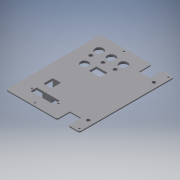
# Autodesk Inventor part: vrch2
Saved by Autodesk Inventor 2016 (Build 200138000, 138)
## iProperties
Created: 2015-11-06
Part Number: vrch2
Material: Generic
Document SubType Name: Modeling
Designer: Jufo
Density: 1 g/cm^3
Appearance: Default
Author: Jufo
Autodesk Inventor part; units mm, degrees
ref_plane "YZ Plane" through (0, 0, 0) normal (1, 0, 0) x (0, 1, 0)
ref_plane "XZ Plane" through (0, 0, 0) normal (0, 1, 0) x (-1, 0, 0)
ref_plane "XY Plane" through (0, 0, 0) normal (0, 0, 1) x (1, 0, 0)
sketch "Sketch1" plane through (0, 0, 0) normal (0, 1, 0) x (-1, 0, 0)
  line L0 (8.278, -23.2242) -> (24.278, -23.2242)
  line L1 (24.278, -23.2242) -> (24.278, 3.7758)
  line L2 (24.278, 3.7758) -> (48.278, 3.7758)
  line L3 (48.278, 3.7758) -> (48.278, -23.2242)
  line L4 (48.278, -23.2242) -> (88.278, -23.2242)
  line L5 (48.278, -23.2242) -> (136.1936, -23.2242)
  line L6 (136.1936, -23.2242) -> (136.1936, 142.7758)
  line L7 (136.1936, 142.7758) -> (48.278, 142.7758)
  line L8 (48.278, 142.7758) -> (48.278, 115.7758)
  line L9 (48.278, 115.7758) -> (24.278, 115.7758)
  line L10 (24.278, 115.7758) -> (24.278, 142.7758)
  line L11 (24.278, 142.7758) -> (24.278, 115.7758)
  line L12 (8.278, 142.7758) -> (24.278, 142.7758)
  line L13 (24.278, 142.7758) -> (8.278, 142.7758)
  line L14 (8.278, 142.7758) -> (8.278, -23.2242)
  line L15 (24.278, 3.7758) -> (24.278, -23.2242)
  circle A0 centre (11.278, -20.2242) radius 1.5
  circle A1 centre (11.278, -20.2242) radius 1.5
  circle A2 centre (11.278, 139.7758) radius 1.5
  circle A3 centre (11.278, 139.7758) radius 1.5
  circle A4 centre (91.278, -20.2242) radius 1.5
  circle A5 centre (91.278, -20.2242) radius 1.5
  circle A6 centre (91.278, 139.7758) radius 1.5
  circle A7 centre (91.278, 139.7758) radius 1.5
  line L16 (133.1936, 141.7758) -> (49.278, 141.7758)
  line L17 (49.278, 141.7758) -> (49.278, 114.7758)
  line L18 (49.278, 114.7758) -> (23.278, 114.7758)
  line L19 (23.278, 114.7758) -> (23.278, 141.7758)
  line L20 (8.278, 59.7758) -> (68.278, 59.7758)
  line L21 (133.1936, 141.7758) -> (133.1936, 59.7758)
  line L22 (23.278, 141.7758) -> (9.278, 141.7758)
  line L23 (9.278, 141.7758) -> (9.278, 59.7758)
  line L24 (133.1936, -22.2242) -> (49.278, -22.2242)
  line L25 (49.278, -22.2242) -> (49.278, 4.7758)
  line L26 (49.278, 4.7758) -> (23.278, 4.7758)
  line L27 (23.278, 4.7758) -> (23.278, -22.2242)
  line L28 (133.1936, -22.2242) -> (133.1936, 59.7758)
  line L29 (23.278, -22.2242) -> (9.278, -22.2242)
  line L30 (9.278, -22.2242) -> (9.278, 59.7758)
  point P0 (0, 0)
  point P1 (0, 0)
  dimension "d0" = 24
  dimension "d1" = 16
  dimension "d2" = 87.9156
  dimension "d3" = 166
  dimension "d4" = 3
  dimension "d5" = 27
  dimension "d6" = 1
  dimension "d8" = 1
  dimension "d9" = 1
  dimension "d10" = 1
  dimension "d11" = 1
  constraints: 62 end point, 13 perpendicular, 8 centre point, 6 symmetric about line, 5 point on line, 4 coincident, 3 horizontal, 2 parallel, 1 midpoint, 1 vertical
  measures "d0" distance of L8.end L9.end
  measures "d1" distance of L10.end L12.start
  measures "d2" distance of L6.end L7.end
  measures "d3" distance of L5.end L6.end
  measures "d4" distance between parallel lines of L6 L21
  measures "d5" distance of L7.end L8.end
  measures "d6" distance between parallel lines of L8 L17
  measures "d8" distance between parallel lines of L18 L9
  measures "d9" distance between parallel lines of L19 L10
  measures "d10" distance between parallel lines of L12 L22
  measures "d11" distance between parallel lines of L14 L23
extrude "Extrusion1" add sketch "Sketch1" along normal blind 2 contours L21 L28 L24 L25 L26 L27 L29 L30 L23 L22 L19 L18 L17 L16
sketch "Sketch2" plane through (0, 2, 0) normal (0, 1, 0) x (1, 0, 0)
  line L0 (-6.278, 25.2242) -> (-26.278, 25.2242)
  line L1 (-26.278, 25.2242) -> (-26.278, 2.2242)
  line L2 (-26.278, 2.2242) -> (-46.278, 2.2242)
  line L3 (-46.278, 2.2242) -> (-46.278, 25.2242)
  line L4 (-46.278, 25.2242) -> (-138.2936, 25.2242)
  line L5 (-133.1936, 22.2242) -> (-133.1936, -141.7758) projected
  line L6 (-133.1936, -59.7758) -> (-63.3349, -59.7758)
  line L7 (-138.2936, 25.2242) -> (-138.2936, -59.7758)
  line L8 (-6.278, 25.2242) -> (-6.278, -59.7758)
  line L9 (-9.278, -141.7758) -> (-9.278, 22.2242) projected
  line L10 (-9.278, 22.2242) -> (-23.278, 22.2242) projected
  line L11 (-23.278, 22.2242) -> (-23.278, -4.7758) projected
  line L12 (-23.278, -4.7758) -> (-49.278, -4.7758) projected
  line L13 (-49.278, -4.7758) -> (-49.278, 22.2242) projected
  line L14 (-49.278, 22.2242) -> (-133.1936, 22.2242) projected
  line L15 (-6.278, -144.7758) -> (-26.278, -144.7758)
  line L16 (-26.278, -144.7758) -> (-26.278, -121.7758)
  line L17 (-26.278, -121.7758) -> (-46.278, -121.7758)
  line L18 (-46.278, -121.7758) -> (-46.278, -144.7758)
  line L19 (-46.278, -144.7758) -> (-138.2936, -144.7758)
  line L20 (-6.278, -144.7758) -> (-6.278, -59.7758)
  line L21 (-138.2936, 25.2242) -> (-138.2936, -144.7758)
  circle A0 centre (-91.278, 20.2242) radius 1.5 projected
  circle A1 centre (-91.278, 20.2242) radius 1.5
  circle A2 centre (-91.278, -139.7758) radius 1.5 projected
  circle A3 centre (-91.278, -139.7758) radius 1.5
  circle A4 centre (-11.278, -139.7758) radius 1.5 projected
  circle A5 centre (-11.278, -139.7758) radius 1.5
  circle A6 centre (-11.278, 20.2242) radius 1.5
  point P0 (0, 0)
  dimension "d14" = 3
  dimension "d15" = 3
  dimension "d16" = 3
  dimension "d17" = 7
  dimension "d18" = 3
  dimension "d19" = 3
  dimension "d130" = 5.1
  constraints: 30 end point, 6 symmetric about line, 5 point on line, 4 centre point, 4 perpendicular, 3 coincident, 2 horizontal, 1 concentric, 1 midpoint, 1 parallel, 1 vertical
  measures "d14" distance between parallel lines of L8 L9
  measures "d15" distance between parallel lines of L0 L10
  measures "d16" distance between parallel lines of L1 L11
  measures "d17" distance between parallel lines of L12 L2
  measures "d18" distance between parallel lines of L13 L3
  measures "d19" distance between parallel lines of L4 L14
  measures "d130" distance between parallel lines of L5 L21
extrude "Extrusion2" add sketch "Sketch2" along normal blind 2
sketch "Sketch9" plane through (0, 4, 0) normal (0, 1, 0) x (1, 0, 0)
  line L0 (-26.278, -121.7758) -> (-6.278, -121.7758)
  line L1 (-6.278, -144.7758) -> (-6.278, 25.2242) projected
  line L2 (-26.278, 2.2242) -> (-6.278, 2.2242)
  line L3 (-16.278, -121.7758) -> (-16.278, -118.7758)
  circle A0 centre (-16.278, -118.7758) radius 3
  line L4 (-16.278, 2.2242) -> (-16.278, -0.7758)
  circle A1 centre (-16.278, -0.7758) radius 3
  line L5 (-81.278, -3.2758) -> (-61.278, -3.2758)
  line L6 (-61.278, -3.2758) -> (-61.278, 10.2242)
  line L7 (-61.278, 10.2242) -> (-81.278, 10.2242)
  line L8 (-81.278, 10.2242) -> (-81.278, -3.2758)
  line L9 (-26.278, 2.2242) -> (-46.278, 2.2242) projected
  line L10 (-26.278, 25.2242) -> (-26.278, 2.2242) projected
  line L11 (-113.628, -102.2758) -> (-99.128, -102.2758)
  line L12 (-99.128, -102.2758) -> (-99.128, -85.2758)
  line L13 (-99.128, -85.2758) -> (-113.628, -85.2758)
  line L14 (-113.628, -85.2758) -> (-113.628, -102.2758)
  circle A2 centre (-115.2936, 3.7242) radius 7
  circle A3 centre (-114.678, -24.7758) radius 7.5
  circle A4 centre (-92.878, -24.7758) radius 7.5
  circle A5 centre (-71.078, -24.7758) radius 7.5
  line L15 (-122.1757, -24.5875) -> (-122.1757, -24.5875)
  line L16 (-100.3757, -24.9641) -> (-100.3757, -24.5875)
  circle A6 centre (-114.678, -39.7758) radius 2.5
  circle A7 centre (-92.878, -39.7758) radius 2.5
  circle A8 centre (-71.078, -39.7758) radius 2.5
  line L17 (-46.278, 25.2242) -> (-138.2936, 25.2242) projected
  line L18 (-49.278, -4.7758) -> (-49.278, 22.2242) projected
  line L19 (-138.2936, 25.2242) -> (-138.2936, -144.7758) projected
  line L20 (-113.628, -125.2758) -> (-72.128, -125.2758)
  line L21 (-72.128, -125.2758) -> (-72.128, -114.2758)
  line L22 (-72.128, -114.2758) -> (-113.628, -114.2758)
  line L23 (-113.628, -114.2758) -> (-113.628, -125.2758)
  line L24 (-46.278, -121.7758) -> (-26.278, -121.7758) projected
  line L25 (-113.628, -119.7758) -> (-116.628, -119.7758)
  circle A9 centre (-116.628, -119.7758) radius 1.5
  line L26 (-72.128, -119.7758) -> (-69.128, -119.7758)
  circle A10 centre (-69.128, -119.7758) radius 1.5
  line L27 (-46.278, -144.7758) -> (-46.278, -121.7758) projected
  line L28 (-65.078, -20.2758) -> (-65.078, -29.2758)
  line L29 (-86.878, -20.2758) -> (-86.878, -29.2758)
  line L30 (-108.678, -20.2758) -> (-108.678, -29.2758)
  arc A11 (-108.678, -29.2758) -> (-108.678, -20.2758) centre (-114.678, -24.7758) ccw
  circle A12 centre (-11.278, 20.2242) radius 1.5 projected
  circle A13 centre (-11.278, -139.7758) radius 1.5 projected
  circle A14 centre (-91.278, -139.7758) radius 1.5 projected
  circle A15 centre (-91.278, 20.2242) radius 1.5 projected
  line L31 (-6.278, 25.2242) -> (-26.278, 25.2242) projected
  line L32 (-26.278, 25.2242) -> (-26.278, 2.2242) projected
  line L33 (-26.278, 2.2242) -> (-46.278, 2.2242) projected
  line L34 (-46.278, 2.2242) -> (-46.278, 25.2242) projected
  line L35 (-46.278, 25.2242) -> (-138.2936, 25.2242) projected
  line L36 (-138.2936, 25.2242) -> (-138.2936, -144.7758) projected
  line L37 (-138.2936, -144.7758) -> (-46.278, -144.7758) projected
  line L38 (-46.278, -144.7758) -> (-46.278, -121.7758) projected
  line L39 (-46.278, -121.7758) -> (-26.278, -121.7758) projected
  line L40 (-26.278, -121.7758) -> (-26.278, -144.7758) projected
  line L41 (-26.278, -144.7758) -> (-6.278, -144.7758) projected
  line L42 (-6.278, -144.7758) -> (-6.278, 25.2242) projected
  point P0 (0, 0)
  point P1 (-99.5314, -28.2373)
  point P2 (-99.5314, -21.3143)
  point P3 (-121.3314, -28.2373)
  point P4 (-121.3314, -21.3143)
  point P5 (-77.7314, -28.2373)
  point P6 (-77.7314, -21.3143)
  dimension "d62" = 3
  dimension "d63" = 6
  dimension "d64" = 3
  dimension "d69" = 20
  dimension "d70" = 17
  dimension "d71" = 14.5
  dimension "d97" = 11
  dimension "d98" = 41.5
  dimension "d99" = 7.5
  dimension "d100" = 3
  dimension "d101" = 3
  dimension "d102" = 3
  dimension "d103" = 3
  dimension "d106" = 25.85
  dimension "d108" = 0
  dimension "d157" = 50
  dimension "d158" = 15
  dimension "d159" = 15
  dimension "d160" = 15
  dimension "d161" = 21.8
  dimension "d162" = 21.8
  dimension "d163" = 15
  dimension "d164" = 15
  dimension "d165" = 15
  dimension "d166" = 50
  dimension "d167" = 50
  dimension "d168" = 15
  dimension "d169" = 6.5
  dimension "d171" = 20
  dimension "d172" = 13.5
  dimension "d173" = 14
  dimension "d174" = 15
  dimension "d175" = 23
  constraints: 46 end point, 18 point on circle, 12 centre point, 9 parallel, 6 horizontal, 5 vertical, 4 coincident, 4 midpoint, 3 perpendicular, 2 point on line, 1 concentric, 1 tangent
  measures "d62" distance of L3.start L3.end
  measures "d63" diameter of A0
  measures "d64" distance of L4.start L4.end
  measures "d69" distance between parallel lines of L1 L10
  measures "d70" distance of L11.end L12.end
  measures "d71" distance of L12.end L13.end
  measures "d97" distance of L20.end L21.end
  measures "d98" distance of L21.end L22.end
  measures "d99" distance between parallel lines of L22 L24
  measures "d100" distance of L25.start L25.end
  measures "d101" diameter of A9
  measures "d102" distance of L26.start L26.end
  measures "d103" diameter of A10
  measures "d106" distance between parallel lines of L27 L21
  measures "d108" distance between parallel lines of L23 L14
  measures "d157" distance from line of A4.centre L17
  measures "d158" distance of A8.centre A5.centre
  measures "d159" distance of A7.centre A4.centre
  measures "d160" distance of A6.centre A3.centre
  measures "d161" distance of A4.centre A3.centre
  measures "d162" distance of A5.centre A4.centre
  measures "d163" diameter of A5
  measures "d164" diameter of A4
  measures "d165" diameter of A3
  measures "d166" distance from line of L35 A5.centre
  measures "d167" distance from line of L17 A3.centre
  measures "d168" distance between parallel lines of L35 L7
  measures "d169" distance from line of L7 A2.centre
  measures "d171" distance of L6.end L7.end
  measures "d172" distance of L5.end L6.end
  measures "d173" diameter of A2
  measures "d174" distance between parallel lines of L34 L6
  measures "d175" distance from line of L19 A2.centre
extrude "Extrusion8" cut sketch "Sketch9" against normal blind 15 contours A0 | A1 | L8 L7 L6 L5 | L14 L13 L12 L11 | A2 | L30 A3 | L29 A4 | L28 A5 | A6 | A7 | A8 | L23 L22 L21 L20 | A9 | A10 picked at (-113.178, -24.7758) picked at (-93.3325, -27.1192) picked at (-69.578, -24.7758)
fillet "Fillet1" radius 3 8 edges at (-46.278, 3, -25.2242) (-26.278, 3, -25.2242) (-6.278, 3, -25.2242) (-6.278, 3, 144.7758) (-46.278, 3, 144.7758) (-26.278, 3, 144.7758) (-138.2936, 3, -25.2242) (-138.2936, 3, 144.7758)
sketch "Sketch10" plane through (0, 0, 0) normal (0, -1, 0) x (1, 0, 0)
  line L0 (-113.628, 85.2758) -> (-113.628, 83.2758)
  line L1 (-113.628, 83.2758) -> (-97.128, 83.2758)
  line L2 (-97.128, 83.2758) -> (-97.128, 104.2758)
  line L3 (-97.128, 104.2758) -> (-113.628, 104.2758)
  line L4 (-113.628, 104.2758) -> (-113.628, 102.2758)
  line L5 (-99.128, 102.2758) -> (-99.128, 85.2758) projected
  line L6 (-113.628, 102.2758) -> (-99.128, 102.2758) projected
  line L7 (-113.628, 85.2758) -> (-99.128, 85.2758)
  line L8 (-99.128, 85.2758) -> (-99.128, 102.2758)
  line L9 (-99.128, 102.2758) -> (-113.628, 102.2758)
  point P0 (0, 0)
  dimension "d112" = 2
  dimension "d113" = 2
  dimension "d114" = 2
  constraints: 16 end point, 5 perpendicular, 1 collinear, 1 horizontal, 1 point on line, 1 vertical
  measures "d112" distance of L0.start L0.end
  measures "d113" distance between parallel lines of L2 L5
  measures "d114" distance between parallel lines of L3 L6
extrude "Extrusion9" add sketch "Sketch10" along normal blind 17
sketch "Sketch11" plane through (0, 0, 0) normal (0, -1, 0) x (1, 0, 0)
  circle A0 centre (-115.2936, -3.7242) radius 7 projected
  line L0 (-112.9685, -17.1192) -> (-110.9685, -17.1192)
  line L1 (-110.9685, -17.1192) -> (-110.9685, -12.2242)
  line L2 (-110.9685, -12.2242) -> (-112.9685, -12.2242)
  line L3 (-114.9685, -12.2242) -> (-114.9685, -17.1192)
  line L4 (-114.9685, -17.1192) -> (-116.9685, -17.1192)
  line L5 (-116.9685, -17.1192) -> (-116.9685, -12.2242)
  line L6 (-116.9685, -12.2242) -> (-114.9685, -12.2242)
  line L7 (-112.9685, -12.2242) -> (-112.9685, -17.1192)
  line L8 (-113.7685, 63.7725) -> (-113.7685, 56.0944)
  arc A1 (-108.678, 29.2758) -> (-108.678, 20.2758) centre (-114.678, 24.7758) ccw projected
  point P0 (0, 0)
  dimension "d117" = 2
  dimension "d118" = 2
  dimension "d120" = 0.8
  dimension "d121" = 1.2
  dimension "d143" = 4.895
  dimension "d146" = 1.525
  dimension "d177" = 8.5
  constraints: 18 end point, 5 perpendicular, 4 point on line, 2 vertical, 1 horizontal
  measures "d117" distance of L1.end L2.end
  measures "d118" distance of L5.end L3.start
  measures "d120" distance between parallel lines of L7 L8
  measures "d121" distance between parallel lines of L8 L3
  measures "d143" distance of L4.end L5.end
  measures "d177" distance from line of A0.centre L6
extrude "Extrusion10" add sketch "Sketch11" along normal blind 8 contours L7 L2 L1 L0 | L3 L4 L5 L6
sketch "Sketch15" plane through (0, 2, 0) normal (0, -1, 0) x (1, 0, 0)
  line L0 (-138.2936, -25.2242) -> (-138.2936, 144.7758) projected
  line L1 (-138.2936, 4.7758) -> (-133.1361, 4.7758)
  line L2 (-138.2936, 114.7758) -> (-133.1361, 114.7758)
  line L3 (-133.1361, 114.7758) -> (-133.1361, 4.7758)
  line L4 (-138.2936, 4.7758) -> (-138.2936, 114.7758)
  line L5 (-49.278, -25.2242) -> (-138.2936, -25.2242) projected
  point P0 (0, 0)
  dimension "d131" = 110
  dimension "d132" = 30
  constraints: 8 end point, 2 horizontal, 2 point on line, 1 collinear, 1 perpendicular
  measures "d131" distance between parallel lines of L1 L2
  measures "d132" distance between parallel lines of L1 L5
extrude "Extrusion12" add sketch "Sketch15" along normal blind 2
sketch "Sketch16" plane through (0, 0, 0) normal (0, -1, 0) x (1, 0, 0)
  circle A0 centre (-115.2936, -3.7242) radius 7 projected
  line L0 (-118.2936, -10.0488) -> (-118.2936, -12.2242)
  line L1 (-118.2936, -12.2242) -> (-112.2936, -12.2242)
  line L2 (-112.2936, -12.2242) -> (-112.2936, -10.0488)
  line L3 (-118.2936, 2.6004) -> (-118.2936, 4.7758)
  line L4 (-118.2936, 4.7758) -> (-112.2936, 4.7758)
  line L5 (-112.2936, 4.7758) -> (-112.2936, 2.6004)
  point P0 (0, 0)
  dimension "d151" = 3
  dimension "d152" = 3
  dimension "d153" = 8.5
  dimension "d154" = 8.5
  constraints: 12 end point, 4 point on circle, 3 perpendicular, 2 vertical
  measures "d151" distance from line of L0 A0.centre
  measures "d152" distance from line of A0.centre L2
  measures "d153" distance from line of L4 A0.centre
  measures "d154" distance from line of A0.centre L1
extrude "Extrusion13" cut sketch "Sketch16" against normal blind 2 contours A0 L3 L4 L5 | L2 L1 L0 A0
equation "\"d104\" = d85"
equation "\"d85\" = 15"
body "Solid1"
